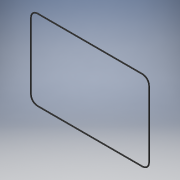
# Autodesk Inventor part: smallgasketback
Saved by Autodesk Inventor 2017 (Build 210142000, 142)
## iProperties
Created: 2017-08-02
Part Number: smallgasketback
Material: Rubber
Document SubType Name: Modeling
Designer: Kai
Density: 0.93 g/cm^3
Appearance: Rubber - Black
Author: Kai
Autodesk Inventor part; units mm, degrees
ref_plane "YZ Plane" through (0, 0, 0) normal (1, 0, 0) x (0, 1, 0)
ref_plane "XZ Plane" through (0, 0, 0) normal (0, 1, 0) x (-1, 0, 0)
ref_plane "XY Plane" through (0, 0, 0) normal (0, 0, 1) x (1, 0, 0)
sketch "Sketch1" plane through (0, 0, 0) normal (0, 0, 1) x (1, 0, 0)
  line L0 (17.78, 0) -> (297.18, 0)
  line L1 (314.96, 17.78) -> (314.96, 195.58)
  line L2 (297.18, 213.36) -> (17.78, 213.36)
  line L3 (0, 195.58) -> (0, 17.78)
  arc A0 (17.78, 213.36) -> (0, 195.58) centre (17.78, 195.58) ccw
  arc A1 (0, 17.78) -> (17.78, 0) centre (17.78, 17.78) ccw
  arc A2 (297.18, 0) -> (314.96, 17.78) centre (297.18, 17.78) ccw
  arc A3 (314.96, 195.58) -> (297.18, 213.36) centre (297.18, 195.58) ccw
  point P0 (0, 0)
  point P1 (314.96, 213.36)
  point P2 (314.96, 0)
  point P3 (0, 213.36)
  dimension "d0" = 314.96
  dimension "d1" = 213.36
  dimension "d2" = 17.78
  constraints: 8 end point, 8 point on circle, 8 point on line, 8 tangent, 4 centre point, 3 equal radius, 2 parallel, 1 horizontal, 1 perpendicular
  measures "d0" distance of point (0, 213.36) point (314.96, 213.36)
  measures "d1" distance of point (314.96, 213.36) point (314.96, 0)
  measures "d2" radius of A0
ref_plane "Work Plane3" through (50.8, 195.58, 0) normal (-1, 0, 0) x (0, -1, 0)
ref_plane "Work Plane2" through (0, 195.58, 0) normal (-1, 0, 0) x (0, -1, 0)
sketch "Sketch2" plane through (50.8, 195.58, 0) normal (-1, 0, 0) x (0, -1, 0)
  circle A0 centre (195.58, 0) radius 1.5875
  dimension "d5" = 3.175
  constraints: 1 centre point, 1 coincident
  measures "d5" diameter of A0
sweep "Sweep1" add profiles "Sketch2" path "Sketch1" path curves L0 A2 L1 A3 L2 A0 L3 A1
ref_plane "Work Plane1" through (0, 195.58, 0) normal (0, 0, 1) x (0, -1, 0)
body "Solid1"
